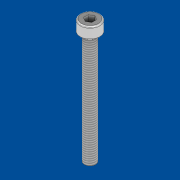
# Autodesk Inventor part: M3-CapScrew
Saved by Autodesk Inventor 2022.2 (Build 262287000, 287)
## iProperties
Created: 2022-02-28
Part Number: M3-CapScrew
Material: 一般
Document SubType Name: Modeling
Designer: Yuta Fujiyama
Density: 1 g/cm^3
Appearance: クローム - つや出し
Author: Yuta Fujiyama
Autodesk Inventor part; units mm, degrees
ref_plane "YZ Plane" through (0, 0, 0) normal (1, 0, 0) x (0, 1, 0)
ref_plane "XZ Plane" through (0, 0, 0) normal (0, 1, 0) x (-1, 0, 0)
ref_plane "XY Plane" through (0, 0, 0) normal (0, 0, 1) x (1, 0, 0)
sketch "スケッチ1" plane through (0, 0, 0) normal (0, 1, 0) x (-1, 0, 0)
  circle A0 centre (0, 0) radius 3.5
  dimension "d0" = 7
  constraints: 1 centre point, 1 coincident
  measures "d0" diameter of A0
extrude "押し出し1" add sketch "スケッチ1" along normal blind 4
sketch "スケッチ2" plane through (0, 0, 0) normal (0, -1, 0) x (1, 0, 0)
  circle A0 centre (0, 0) radius 2
  dimension "d3" = 4
  constraints: 1 centre point, 1 coincident
  measures "d3" diameter of A0
extrude "押し出し2" add sketch "スケッチ2" along normal blind 40
fillet "フィレット1" radius 0.5 1 edges at (3.5, 4, 0)
fillet "フィレット1" radius 0.2 1 edges at (3.5, 0, 0)
sketch "スケッチ3" plane through (0, 4, 0) normal (0, 1, 0) x (1, 0, 0)
  line L0 (0, 1.7321) -> (-1.5, 0.866)
  line L1 (-1.5, 0.866) -> (-1.5, -0.866)
  line L2 (-1.5, -0.866) -> (0, -1.7321)
  line L3 (0, -1.7321) -> (1.5, -0.866)
  line L4 (1.5, -0.866) -> (1.5, 0.866)
  line L5 (1.5, 0.866) -> (0, 1.7321)
  line L6 (0, 1.7321) -> (0, -1.7321) construction
  circle A0 centre (0, 0) radius 1.7321 construction
  dimension "d12" = 3
  constraints: 14 end point, 5 point on circle, 3 equal length, 2 coincident, 1 centre point, 1 midpoint, 1 parallel, 1 vertical
  measures "d12" distance between parallel lines of L4 L1
extrude "押し出し3" cut sketch "スケッチ3" against normal blind 2
thread "ねじ1" size "M4x0.7" class "6g" standard "ANSI Metric M Profile" full length
